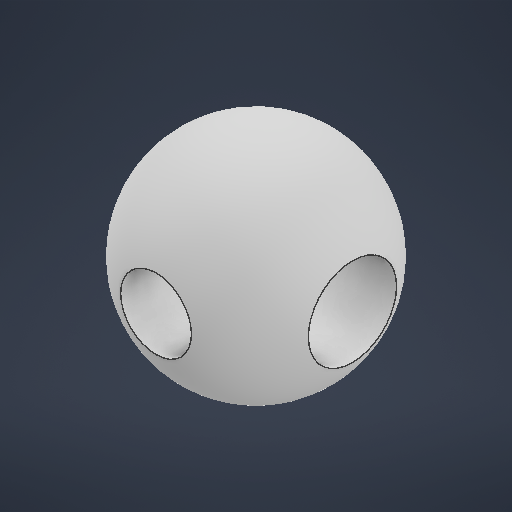
# Autodesk Inventor part: parca7
Saved by Autodesk Inventor 2025.4 (Build 294407000, 407)
## iProperties
Created: 2026-06-20
Part Number: parca7
Material: Generic
Document SubType Name: Modeling
Designer: yigithan
Density: 1 g/cm^3
Appearance: Default
Author: yigithan
Autodesk Inventor part; units mm, degrees
ref_plane "YZ Plane" through (0, 0, 0) normal (1, 0, 0) x (0, 1, 0)
ref_plane "XZ Plane" through (0, 0, 0) normal (0, 1, 0) x (-1, 0, 0)
ref_plane "XY Plane" through (0, 0, 0) normal (0, 0, 1) x (1, 0, 0)
sketch "Sketch1" plane through (0, 0, 0) normal (0, 0, 1) x (1, 0, 0)
  arc A0 (8.6683, 3.96) -> (-8.6683, 3.96) centre (0, 0) ccw
  line L0 (-8.6683, 3.96) -> (8.6683, 3.96)
  line L1 (-16.3329, 0) -> (13.8423, 0)
  dimension "d0" = 19.06
  constraints: 4 end point, 2 horizontal, 2 point on circle, 1 centre point, 1 coincident
  measures "d0" diameter of A0
revolve "Revolution1" add sketch "Sketch1" angle 360 about axis through (-16.3329, 0, 0) along (1, 0, 0)
sketch "Sketch2" plane through (0, 0, 0) normal (0, 0, 1) x (1, 0, 0)
  circle A0 centre (0, 0) radius 3.18
  dimension "d4" = 6.36
  constraints: 1 centre point, 1 coincident
  measures "d4" diameter of A0
extrude "Extrusion1" cut sketch "Sketch2" along normal mid plane 23.5
body "Solid1"
